Autodesk Fusion 360 part; units mm, degrees
(part 4 of 13)
sketch "Sketch30" plane through (0, 0, 9) normal (0, 0, 1) x (-1, 0, 0)
  line L0 (-20, -24.98) -> (-20, -25.98)
  line L1 (-20, -25.98) -> (-21, -25.98)
  line L2 (-21, -25.98) -> (-21, -24.98)
  line L3 (-21, -24.98) -> (-20, -24.98)
  line L4 (-23, -24.98) -> (-23, -25.98)
  line L5 (-23, -25.98) -> (-24, -25.98)
  line L6 (-24, -25.98) -> (-24, -24.98)
  line L7 (-24, -24.98) -> (-23, -24.98)
  line L8 (-20, -27.61) -> (-20, -28.61)
  line L9 (-20, -28.61) -> (-21, -28.61)
  line L10 (-21, -28.61) -> (-21, -27.61)
  line L11 (-21, -27.61) -> (-20, -27.61)
  line L12 (-23, -27.61) -> (-23, -28.61)
  line L13 (-23, -28.61) -> (-24, -28.61)
  line L14 (-24, -28.61) -> (-24, -27.61)
  line L15 (-24, -27.61) -> (-23, -27.61)
  line L16 (-20, -30.24) -> (-20, -31.24)
  line L17 (-20, -31.24) -> (-21, -31.24)
  line L18 (-21, -31.24) -> (-21, -30.24)
  line L19 (-21, -30.24) -> (-20, -30.24)
  line L20 (-23, -30.24) -> (-23, -31.24)
  line L21 (-23, -31.24) -> (-24, -31.24)
  line L22 (-24, -31.24) -> (-24, -30.24)
  line L23 (-24, -30.24) -> (-23, -30.24)
  line L24 (-20, -32.87) -> (-20, -33.87)
  line L25 (-20, -33.87) -> (-21, -33.87)
  line L26 (-21, -33.87) -> (-21, -32.87)
  line L27 (-21, -32.87) -> (-20, -32.87)
  line L28 (-23, -32.87) -> (-23, -33.87)
  line L29 (-23, -33.87) -> (-24, -33.87)
  line L30 (-24, -33.87) -> (-24, -32.87)
  line L31 (-24, -32.87) -> (-23, -32.87)
  line L32 (-20, -35.5) -> (-20, -36.5)
  line L33 (-20, -36.5) -> (-21, -36.5)
  line L34 (-21, -36.5) -> (-21, -35.5)
  line L35 (-21, -35.5) -> (-20, -35.5)
  line L36 (-23, -35.5) -> (-23, -36.5)
  line L37 (-23, -36.5) -> (-24, -36.5)
  line L38 (-24, -36.5) -> (-24, -35.5)
  line L39 (-24, -35.5) -> (-23, -35.5)
  line L40 (-13.7, 38.77) -> (-13.7, 37.77)
  line L41 (-13.7, 37.77) -> (-14.7, 37.77)
  line L42 (-14.7, 37.77) -> (-14.7, 38.77)
  line L43 (-14.7, 38.77) -> (-13.7, 38.77)
  line L44 (-13.7, 36.14) -> (-13.7, 35.14)
  line L45 (-13.7, 35.14) -> (-14.7, 35.14)
  line L46 (-14.7, 35.14) -> (-14.7, 36.14)
  line L47 (-14.7, 36.14) -> (-13.7, 36.14)
  line L48 (-13.7, 33.51) -> (-13.7, 32.51)
  line L49 (-13.7, 32.51) -> (-14.7, 32.51)
  line L50 (-14.7, 32.51) -> (-14.7, 33.51)
  line L51 (-14.7, 33.51) -> (-13.7, 33.51)
  line L52 (-13.7, 30.88) -> (-13.7, 29.88)
  line L53 (-13.7, 29.88) -> (-14.7, 29.88)
  line L54 (-14.7, 29.88) -> (-14.7, 30.88)
  line L55 (-14.7, 30.88) -> (-13.7, 30.88)
  line L56 (-13.7, 28.25) -> (-13.7, 27.25)
  line L57 (-13.7, 27.25) -> (-14.7, 27.25)
  line L58 (-14.7, 27.25) -> (-14.7, 28.25)
  line L59 (-14.7, 28.25) -> (-13.7, 28.25)
  line L60 (-13.7, 25.62) -> (-13.7, 24.62)
  line L61 (-13.7, 24.62) -> (-14.7, 24.62)
  line L62 (-14.7, 24.62) -> (-14.7, 25.62)
  line L63 (-14.7, 25.62) -> (-13.7, 25.62)
  line L64 (-13.7, 22.99) -> (-13.7, 21.99)
  line L65 (-13.7, 21.99) -> (-14.7, 21.99)
  line L66 (-14.7, 21.99) -> (-14.7, 22.99)
  line L67 (-14.7, 22.99) -> (-13.7, 22.99)
  line L68 (-13.7, 20.36) -> (-13.7, 19.36)
  line L69 (-13.7, 19.36) -> (-14.7, 19.36)
  line L70 (-14.7, 19.36) -> (-14.7, 20.36)
  line L71 (-14.7, 20.36) -> (-13.7, 20.36)
  line L72 (-13.7, 17.73) -> (-13.7, 16.73)
  line L73 (-13.7, 16.73) -> (-14.7, 16.73)
  line L74 (-14.7, 16.73) -> (-14.7, 17.73)
  line L75 (-14.7, 17.73) -> (-13.7, 17.73)
  line L76 (-13.7, 15.1) -> (-13.7, 14.1)
  line L77 (-13.7, 14.1) -> (-14.7, 14.1)
  line L78 (-14.7, 14.1) -> (-14.7, 15.1)
  line L79 (-14.7, 15.1) -> (-13.7, 15.1)
  line L80 (-13.7, 12.47) -> (-13.7, 11.47)
  line L81 (-13.7, 11.47) -> (-14.7, 11.47)
  line L82 (-14.7, 11.47) -> (-14.7, 12.47)
  line L83 (-14.7, 12.47) -> (-13.7, 12.47)
  line L84 (-13.7, 9.84) -> (-13.7, 8.84)
  line L85 (-13.7, 8.84) -> (-14.7, 8.84)
  line L86 (-14.7, 8.84) -> (-14.7, 9.84)
  line L87 (-14.7, 9.84) -> (-13.7, 9.84)
  line L88 (-13.7, 7.21) -> (-13.7, 6.21)
  line L89 (-13.7, 6.21) -> (-14.7, 6.21)
  line L90 (-14.7, 6.21) -> (-14.7, 7.21)
  line L91 (-14.7, 7.21) -> (-13.7, 7.21)
  line L92 (-13.7, 4.58) -> (-13.7, 3.58)
  line L93 (-13.7, 3.58) -> (-14.7, 3.58)
  line L94 (-14.7, 3.58) -> (-14.7, 4.58)
  line L95 (-14.7, 4.58) -> (-13.7, 4.58)
  line L96 (-13.7, 1.95) -> (-13.7, 0.95)
  line L97 (-13.7, 0.95) -> (-14.7, 0.95)
  line L98 (-14.7, 0.95) -> (-14.7, 1.95)
  line L99 (-14.7, 1.95) -> (-13.7, 1.95)
  line L100 (-13.7, -0.68) -> (-13.7, -1.68)
  line L101 (-13.7, -1.68) -> (-14.7, -1.68)
  line L102 (-14.7, -1.68) -> (-14.7, -0.68)
  line L103 (-14.7, -0.68) -> (-13.7, -0.68)
  line L104 (-13.7, -3.31) -> (-13.7, -4.31)
  line L105 (-13.7, -4.31) -> (-14.7, -4.31)
  line L106 (-14.7, -4.31) -> (-14.7, -3.31)
  line L107 (-14.7, -3.31) -> (-13.7, -3.31)
  line L108 (-13.7, -5.94) -> (-13.7, -6.94)
  line L109 (-13.7, -6.94) -> (-14.7, -6.94)
  line L110 (-14.7, -6.94) -> (-14.7, -5.94)
  line L111 (-14.7, -5.94) -> (-13.7, -5.94)
  line L112 (-13.7, -8.57) -> (-13.7, -9.57)
  line L113 (-13.7, -9.57) -> (-14.7, -9.57)
  line L114 (-14.7, -9.57) -> (-14.7, -8.57)
  line L115 (-14.7, -8.57) -> (-13.7, -8.57)
  line L116 (-13.7, -11.2) -> (-13.7, -12.2)
  line L117 (-13.7, -12.2) -> (-14.7, -12.2)
  line L118 (-14.7, -12.2) -> (-14.7, -11.2)
  line L119 (-14.7, -11.2) -> (-13.7, -11.2)
  line L120 (-13.7, -13.83) -> (-13.7, -14.83)
  line L121 (-13.7, -14.83) -> (-14.7, -14.83)
  line L122 (-14.7, -14.83) -> (-14.7, -13.83)
  line L123 (-14.7, -13.83) -> (-13.7, -13.83)
  line L124 (-13.7, -16.46) -> (-13.7, -17.46)
  line L125 (-13.7, -17.46) -> (-14.7, -17.46)
  line L126 (-14.7, -17.46) -> (-14.7, -16.46)
  line L127 (-14.7, -16.46) -> (-13.7, -16.46)
  line L128 (-13.7, -19.09) -> (-13.7, -20.09)
  line L129 (-13.7, -20.09) -> (-14.7, -20.09)
  line L130 (-14.7, -20.09) -> (-14.7, -19.09)
  line L131 (-14.7, -19.09) -> (-13.7, -19.09)
  line L132 (-13.7, -21.72) -> (-13.7, -22.72)
  line L133 (-13.7, -22.72) -> (-14.7, -22.72)
  line L134 (-14.7, -22.72) -> (-14.7, -21.72)
  line L135 (-14.7, -21.72) -> (-13.7, -21.72)
  line L136 (-13.7, -24.35) -> (-13.7, -25.35)
  line L137 (-13.7, -25.35) -> (-14.7, -25.35)
  line L138 (-14.7, -25.35) -> (-14.7, -24.35)
  line L139 (-14.7, -24.35) -> (-13.7, -24.35)
  line L140 (-13.7, -26.98) -> (-13.7, -27.98)
  line L141 (-13.7, -27.98) -> (-14.7, -27.98)
  line L142 (-14.7, -27.98) -> (-14.7, -26.98)
  line L143 (-14.7, -26.98) -> (-13.7, -26.98)
  line L144 (-13.7, -29.61) -> (-13.7, -30.61)
  line L145 (-13.7, -30.61) -> (-14.7, -30.61)
  line L146 (-14.7, -30.61) -> (-14.7, -29.61)
  line L147 (-14.7, -29.61) -> (-13.7, -29.61)
  line L148 (-13.7, -32.24) -> (-13.7, -33.24)
  line L149 (-13.7, -33.24) -> (-14.7, -33.24)
  line L150 (-14.7, -33.24) -> (-14.7, -32.24)
  line L151 (-14.7, -32.24) -> (-13.7, -32.24)
  line L152 (-13.7, -34.87) -> (-13.7, -35.87)
  line L153 (-13.7, -35.87) -> (-14.7, -35.87)
  line L154 (-14.7, -35.87) -> (-14.7, -34.87)
  line L155 (-14.7, -34.87) -> (-13.7, -34.87)
  line L156 (-13.7, -37.5) -> (-13.7, -38.5)
  line L157 (-13.7, -38.5) -> (-14.7, -38.5)
  line L158 (-14.7, -38.5) -> (-14.7, -37.5)
  line L159 (-14.7, -37.5) -> (-13.7, -37.5)
  line L160 (-10.9, 38.77) -> (-10.9, 37.77)
  line L161 (-10.9, 37.77) -> (-11.9, 37.77)
  line L162 (-11.9, 37.77) -> (-11.9, 38.77)
  line L163 (-11.9, 38.77) -> (-10.9, 38.77)
  line L164 (-10.9, 36.14) -> (-10.9, 35.14)
  line L165 (-10.9, 35.14) -> (-11.9, 35.14)
  line L166 (-11.9, 35.14) -> (-11.9, 36.14)
  line L167 (-11.9, 36.14) -> (-10.9, 36.14)
  line L168 (-10.9, 33.51) -> (-10.9, 32.51)
  line L169 (-10.9, 32.51) -> (-11.9, 32.51)
  line L170 (-11.9, 32.51) -> (-11.9, 33.51)
  line L171 (-11.9, 33.51) -> (-10.9, 33.51)
  line L172 (-10.9, 30.88) -> (-10.9, 29.88)
  line L173 (-10.9, 29.88) -> (-11.9, 29.88)
  line L174 (-11.9, 29.88) -> (-11.9, 30.88)
  line L175 (-11.9, 30.88) -> (-10.9, 30.88)
  line L176 (-10.9, 28.25) -> (-10.9, 27.25)
  line L177 (-10.9, 27.25) -> (-11.9, 27.25)
  line L178 (-11.9, 27.25) -> (-11.9, 28.25)
  line L179 (-11.9, 28.25) -> (-10.9, 28.25)
  line L180 (-10.9, 25.62) -> (-10.9, 24.62)
  line L181 (-10.9, 24.62) -> (-11.9, 24.62)
  line L182 (-11.9, 24.62) -> (-11.9, 25.62)
  line L183 (-11.9, 25.62) -> (-10.9, 25.62)
  line L184 (-10.9, 22.99) -> (-10.9, 21.99)
  line L185 (-10.9, 21.99) -> (-11.9, 21.99)
  line L186 (-11.9, 21.99) -> (-11.9, 22.99)
  line L187 (-11.9, 22.99) -> (-10.9, 22.99)
  line L188 (-10.9, 20.36) -> (-10.9, 19.36)
  line L189 (-10.9, 19.36) -> (-11.9, 19.36)
  line L190 (-11.9, 19.36) -> (-11.9, 20.36)
  line L191 (-11.9, 20.36) -> (-10.9, 20.36)
  line L192 (-10.9, 17.73) -> (-10.9, 16.73)
  line L193 (-10.9, 16.73) -> (-11.9, 16.73)
  line L194 (-11.9, 16.73) -> (-11.9, 17.73)
  line L195 (-11.9, 17.73) -> (-10.9, 17.73)
  line L196 (-10.9, 15.1) -> (-10.9, 14.1)
  line L197 (-10.9, 14.1) -> (-11.9, 14.1)
  line L198 (-11.9, 14.1) -> (-11.9, 15.1)
  line L199 (-11.9, 15.1) -> (-10.9, 15.1)
  line L200 (-10.9, 12.47) -> (-10.9, 11.47)
  line L201 (-10.9, 11.47) -> (-11.9, 11.47)
  line L202 (-11.9, 11.47) -> (-11.9, 12.47)
  line L203 (-11.9, 12.47) -> (-10.9, 12.47)
  line L204 (-10.9, 9.84) -> (-10.9, 8.84)
  line L205 (-10.9, 8.84) -> (-11.9, 8.84)
  line L206 (-11.9, 8.84) -> (-11.9, 9.84)
  line L207 (-11.9, 9.84) -> (-10.9, 9.84)
  line L208 (-10.9, 7.21) -> (-10.9, 6.21)
  line L209 (-10.9, 6.21) -> (-11.9, 6.21)
  line L210 (-11.9, 6.21) -> (-11.9, 7.21)
  line L211 (-11.9, 7.21) -> (-10.9, 7.21)
  line L212 (-10.9, 4.58) -> (-10.9, 3.58)
  line L213 (-10.9, 3.58) -> (-11.9, 3.58)
  line L214 (-11.9, 3.58) -> (-11.9, 4.58)
  line L215 (-11.9, 4.58) -> (-10.9, 4.58)
  line L216 (-10.9, 1.95) -> (-10.9, 0.95)
  line L217 (-10.9, 0.95) -> (-11.9, 0.95)
  line L218 (-11.9, 0.95) -> (-11.9, 1.95)
  line L219 (-11.9, 1.95) -> (-10.9, 1.95)
  line L220 (-10.9, -0.68) -> (-10.9, -1.68)
  line L221 (-10.9, -1.68) -> (-11.9, -1.68)
  line L222 (-11.9, -1.68) -> (-11.9, -0.68)
  line L223 (-11.9, -0.68) -> (-10.9, -0.68)
  line L224 (-10.9, -3.31) -> (-10.9, -4.31)
  line L225 (-10.9, -4.31) -> (-11.9, -4.31)
  line L226 (-11.9, -4.31) -> (-11.9, -3.31)
  line L227 (-11.9, -3.31) -> (-10.9, -3.31)
  line L228 (-10.9, -5.94) -> (-10.9, -6.94)
  line L229 (-10.9, -6.94) -> (-11.9, -6.94)
  line L230 (-11.9, -6.94) -> (-11.9, -5.94)
  line L231 (-11.9, -5.94) -> (-10.9, -5.94)
  line L232 (-10.9, -8.57) -> (-10.9, -9.57)
  line L233 (-10.9, -9.57) -> (-11.9, -9.57)
  line L234 (-11.9, -9.57) -> (-11.9, -8.57)
  line L235 (-11.9, -8.57) -> (-10.9, -8.57)
  line L236 (-10.9, -11.2) -> (-10.9, -12.2)
  line L237 (-10.9, -12.2) -> (-11.9, -12.2)
  line L238 (-11.9, -12.2) -> (-11.9, -11.2)
  line L239 (-11.9, -11.2) -> (-10.9, -11.2)
  line L240 (-10.9, -13.83) -> (-10.9, -14.83)
  line L241 (-10.9, -14.83) -> (-11.9, -14.83)
  line L242 (-11.9, -14.83) -> (-11.9, -13.83)
  line L243 (-11.9, -13.83) -> (-10.9, -13.83)
  line L244 (-10.9, -16.46) -> (-10.9, -17.46)
  line L245 (-10.9, -17.46) -> (-11.9, -17.46)
  line L246 (-11.9, -17.46) -> (-11.9, -16.46)
  line L247 (-11.9, -16.46) -> (-10.9, -16.46)
  line L248 (-10.9, -19.09) -> (-10.9, -20.09)
  line L249 (-10.9, -20.09) -> (-11.9, -20.09)
  line L250 (-11.9, -20.09) -> (-11.9, -19.09)
  line L251 (-11.9, -19.09) -> (-10.9, -19.09)
  line L252 (-10.9, -21.72) -> (-10.9, -22.72)
  line L253 (-10.9, -22.72) -> (-11.9, -22.72)
  line L254 (-11.9, -22.72) -> (-11.9, -21.72)
  line L255 (-11.9, -21.72) -> (-10.9, -21.72)
  line L256 (-10.9, -24.35) -> (-10.9, -25.35)
  line L257 (-10.9, -25.35) -> (-11.9, -25.35)
  line L258 (-11.9, -25.35) -> (-11.9, -24.35)
  line L259 (-11.9, -24.35) -> (-10.9, -24.35)
  line L260 (-10.9, -26.98) -> (-10.9, -27.98)
  line L261 (-10.9, -27.98) -> (-11.9, -27.98)
  line L262 (-11.9, -27.98) -> (-11.9, -26.98)
  line L263 (-11.9, -26.98) -> (-10.9, -26.98)
  line L264 (-10.9, -29.61) -> (-10.9, -30.61)
  line L265 (-10.9, -30.61) -> (-11.9, -30.61)
  line L266 (-11.9, -30.61) -> (-11.9, -29.61)
  line L267 (-11.9, -29.61) -> (-10.9, -29.61)
  line L268 (-10.9, -32.24) -> (-10.9, -33.24)
  line L269 (-10.9, -33.24) -> (-11.9, -33.24)
  line L270 (-11.9, -33.24) -> (-11.9, -32.24)
  line L271 (-11.9, -32.24) -> (-10.9, -32.24)
  line L272 (-10.9, -34.87) -> (-10.9, -35.87)
  line L273 (-10.9, -35.87) -> (-11.9, -35.87)
  line L274 (-11.9, -35.87) -> (-11.9, -34.87)
  line L275 (-11.9, -34.87) -> (-10.9, -34.87)
  line L276 (-10.9, -37.5) -> (-10.9, -38.5)
  line L277 (-10.9, -38.5) -> (-11.9, -38.5)
  line L278 (-11.9, -38.5) -> (-11.9, -37.5)
  line L279 (-11.9, -37.5) -> (-10.9, -37.5)
  line L280 (-8.1, 38.77) -> (-8.1, 37.77)
  line L281 (-8.1, 37.77) -> (-9.1, 37.77)
  line L282 (-9.1, 37.77) -> (-9.1, 38.77)
  line L283 (-9.1, 38.77) -> (-8.1, 38.77)
  line L284 (-8.1, 36.14) -> (-8.1, 35.14)
  line L285 (-8.1, 35.14) -> (-9.1, 35.14)
  line L286 (-9.1, 35.14) -> (-9.1, 36.14)
  line L287 (-9.1, 36.14) -> (-8.1, 36.14)
  line L288 (-8.1, 33.51) -> (-8.1, 32.51)
  line L289 (-8.1, 32.51) -> (-9.1, 32.51)
  line L290 (-9.1, 32.51) -> (-9.1, 33.51)
  line L291 (-9.1, 33.51) -> (-8.1, 33.51)
  line L292 (-8.1, 30.88) -> (-8.1, 29.88)
  line L293 (-8.1, 29.88) -> (-9.1, 29.88)
  line L294 (-9.1, 29.88) -> (-9.1, 30.88)
  line L295 (-9.1, 30.88) -> (-8.1, 30.88)
  line L296 (-8.1, 28.25) -> (-8.1, 27.25)
  line L297 (-8.1, 27.25) -> (-9.1, 27.25)
  line L298 (-9.1, 27.25) -> (-9.1, 28.25)
  line L299 (-9.1, 28.25) -> (-8.1, 28.25)
  line L300 (-8.1, 25.62) -> (-8.1, 24.62)
  line L301 (-8.1, 24.62) -> (-9.1, 24.62)
  line L302 (-9.1, 24.62) -> (-9.1, 25.62)
  line L303 (-9.1, 25.62) -> (-8.1, 25.62)
  line L304 (-8.1, 22.99) -> (-8.1, 21.99)
  line L305 (-8.1, 21.99) -> (-9.1, 21.99)
  line L306 (-9.1, 21.99) -> (-9.1, 22.99)
  line L307 (-9.1, 22.99) -> (-8.1, 22.99)
  line L308 (-8.1, 20.36) -> (-8.1, 19.36)
  line L309 (-8.1, 19.36) -> (-9.1, 19.36)
  line L310 (-9.1, 19.36) -> (-9.1, 20.36)
  line L311 (-9.1, 20.36) -> (-8.1, 20.36)
  line L312 (-8.1, 17.73) -> (-8.1, 16.73)
  line L313 (-8.1, 16.73) -> (-9.1, 16.73)
  line L314 (-9.1, 16.73) -> (-9.1, 17.73)
  line L315 (-9.1, 17.73) -> (-8.1, 17.73)
  line L316 (-8.1, 15.1) -> (-8.1, 14.1)
  line L317 (-8.1, 14.1) -> (-9.1, 14.1)
  line L318 (-9.1, 14.1) -> (-9.1, 15.1)
  line L319 (-9.1, 15.1) -> (-8.1, 15.1)
  line L320 (-8.1, 12.47) -> (-8.1, 11.47)
  line L321 (-8.1, 11.47) -> (-9.1, 11.47)
  line L322 (-9.1, 11.47) -> (-9.1, 12.47)
  line L323 (-9.1, 12.47) -> (-8.1, 12.47)
  line L324 (-8.1, 9.84) -> (-8.1, 8.84)
  line L325 (-8.1, 8.84) -> (-9.1, 8.84)
  line L326 (-9.1, 8.84) -> (-9.1, 9.84)
  line L327 (-9.1, 9.84) -> (-8.1, 9.84)
  line L328 (-8.1, 7.21) -> (-8.1, 6.21)
  line L329 (-8.1, 6.21) -> (-9.1, 6.21)
  line L330 (-9.1, 6.21) -> (-9.1, 7.21)
  line L331 (-9.1, 7.21) -> (-8.1, 7.21)
  line L332 (-8.1, 4.58) -> (-8.1, 3.58)
  line L333 (-8.1, 3.58) -> (-9.1, 3.58)
  line L334 (-9.1, 3.58) -> (-9.1, 4.58)
  line L335 (-9.1, 4.58) -> (-8.1, 4.58)
  line L336 (-8.1, 1.95) -> (-8.1, 0.95)
  line L337 (-8.1, 0.95) -> (-9.1, 0.95)
  line L338 (-9.1, 0.95) -> (-9.1, 1.95)
  line L339 (-9.1, 1.95) -> (-8.1, 1.95)
  line L340 (-8.1, -0.68) -> (-8.1, -1.68)
  line L341 (-8.1, -1.68) -> (-9.1, -1.68)
  line L342 (-9.1, -1.68) -> (-9.1, -0.68)
  line L343 (-9.1, -0.68) -> (-8.1, -0.68)
  line L344 (-8.1, -3.31) -> (-8.1, -4.31)
  line L345 (-8.1, -4.31) -> (-9.1, -4.31)
  line L346 (-9.1, -4.31) -> (-9.1, -3.31)
  line L347 (-9.1, -3.31) -> (-8.1, -3.31)
  line L348 (-8.1, -5.94) -> (-8.1, -6.94)
  line L349 (-8.1, -6.94) -> (-9.1, -6.94)
  line L350 (-9.1, -6.94) -> (-9.1, -5.94)
  line L351 (-9.1, -5.94) -> (-8.1, -5.94)
  line L352 (-8.1, -8.57) -> (-8.1, -9.57)
  line L353 (-8.1, -9.57) -> (-9.1, -9.57)
  line L354 (-9.1, -9.57) -> (-9.1, -8.57)
  line L355 (-9.1, -8.57) -> (-8.1, -8.57)
  line L356 (-8.1, -11.2) -> (-8.1, -12.2)
  line L357 (-8.1, -12.2) -> (-9.1, -12.2)
  line L358 (-9.1, -12.2) -> (-9.1, -11.2)
  line L359 (-9.1, -11.2) -> (-8.1, -11.2)
  line L360 (-8.1, -13.83) -> (-8.1, -14.83)
  line L361 (-8.1, -14.83) -> (-9.1, -14.83)
  line L362 (-9.1, -14.83) -> (-9.1, -13.83)
  line L363 (-9.1, -13.83) -> (-8.1, -13.83)
  line L364 (-8.1, -16.46) -> (-8.1, -17.46)
  line L365 (-8.1, -17.46) -> (-9.1, -17.46)
  line L366 (-9.1, -17.46) -> (-9.1, -16.46)
  line L367 (-9.1, -16.46) -> (-8.1, -16.46)
  line L368 (-8.1, -19.09) -> (-8.1, -20.09)
  line L369 (-8.1, -20.09) -> (-9.1, -20.09)
  line L370 (-9.1, -20.09) -> (-9.1, -19.09)
  line L371 (-9.1, -19.09) -> (-8.1, -19.09)
  line L372 (-8.1, -21.72) -> (-8.1, -22.72)
  line L373 (-8.1, -22.72) -> (-9.1, -22.72)
  line L374 (-9.1, -22.72) -> (-9.1, -21.72)
  line L375 (-9.1, -21.72) -> (-8.1, -21.72)
  line L376 (-8.1, -24.35) -> (-8.1, -25.35)
  line L377 (-8.1, -25.35) -> (-9.1, -25.35)
  line L378 (-9.1, -25.35) -> (-9.1, -24.35)
  line L379 (-9.1, -24.35) -> (-8.1, -24.35)
  line L380 (-8.1, -26.98) -> (-8.1, -27.98)
  line L381 (-8.1, -27.98) -> (-9.1, -27.98)
  line L382 (-9.1, -27.98) -> (-9.1, -26.98)
  line L383 (-9.1, -26.98) -> (-8.1, -26.98)
  line L384 (-8.1, -29.61) -> (-8.1, -30.61)
  line L385 (-8.1, -30.61) -> (-9.1, -30.61)
  line L386 (-9.1, -30.61) -> (-9.1, -29.61)
  line L387 (-9.1, -29.61) -> (-8.1, -29.61)
  line L388 (-8.1, -32.24) -> (-8.1, -33.24)
  line L389 (-8.1, -33.24) -> (-9.1, -33.24)
  line L390 (-9.1, -33.24) -> (-9.1, -32.24)
  line L391 (-9.1, -32.24) -> (-8.1, -32.24)
  line L392 (-8.1, -34.87) -> (-8.1, -35.87)
  line L393 (-8.1, -35.87) -> (-9.1, -35.87)
  line L394 (-9.1, -35.87) -> (-9.1, -34.87)
  line L395 (-9.1, -34.87) -> (-8.1, -34.87)
  line L396 (-8.1, -37.5) -> (-8.1, -38.5)
  line L397 (-8.1, -38.5) -> (-9.1, -38.5)
  line L398 (-9.1, -38.5) -> (-9.1, -37.5)
  line L399 (-9.1, -37.5) -> (-8.1, -37.5)
  line L400 (-5.3, 38.77) -> (-5.3, 37.77)
  line L401 (-5.3, 37.77) -> (-6.3, 37.77)
  line L402 (-6.3, 37.77) -> (-6.3, 38.77)
  line L403 (-6.3, 38.77) -> (-5.3, 38.77)
  line L404 (-5.3, 36.14) -> (-5.3, 35.14)
  line L405 (-5.3, 35.14) -> (-6.3, 35.14)
  line L406 (-6.3, 35.14) -> (-6.3, 36.14)
  line L407 (-6.3, 36.14) -> (-5.3, 36.14)
  line L408 (-5.3, 33.51) -> (-5.3, 32.51)
  line L409 (-5.3, 32.51) -> (-6.3, 32.51)
  line L410 (-6.3, 32.51) -> (-6.3, 33.51)
  line L411 (-6.3, 33.51) -> (-5.3, 33.51)
  line L412 (-5.3, 30.88) -> (-5.3, 29.88)
  line L413 (-5.3, 29.88) -> (-6.3, 29.88)
  line L414 (-6.3, 29.88) -> (-6.3, 30.88)
  line L415 (-6.3, 30.88) -> (-5.3, 30.88)
  line L416 (-5.3, 28.25) -> (-5.3, 27.25)
  line L417 (-5.3, 27.25) -> (-6.3, 27.25)
  line L418 (-6.3, 27.25) -> (-6.3, 28.25)
  line L419 (-6.3, 28.25) -> (-5.3, 28.25)
  line L420 (-5.3, 25.62) -> (-5.3, 24.62)
  line L421 (-5.3, 24.62) -> (-6.3, 24.62)
  line L422 (-6.3, 24.62) -> (-6.3, 25.62)
  line L423 (-6.3, 25.62) -> (-5.3, 25.62)
  line L424 (-5.3, 22.99) -> (-5.3, 21.99)
  line L425 (-5.3, 21.99) -> (-6.3, 21.99)
  line L426 (-6.3, 21.99) -> (-6.3, 22.99)
  line L427 (-6.3, 22.99) -> (-5.3, 22.99)
  line L428 (-5.3, 20.36) -> (-5.3, 19.36)
  line L429 (-5.3, 19.36) -> (-6.3, 19.36)
  line L430 (-6.3, 19.36) -> (-6.3, 20.36)
  line L431 (-6.3, 20.36) -> (-5.3, 20.36)
  line L432 (-5.3, 17.73) -> (-5.3, 16.73)
  line L433 (-5.3, 16.73) -> (-6.3, 16.73)
  line L434 (-6.3, 16.73) -> (-6.3, 17.73)
  line L435 (-6.3, 17.73) -> (-5.3, 17.73)
  line L436 (-5.3, 15.1) -> (-5.3, 14.1)
  line L437 (-5.3, 14.1) -> (-6.3, 14.1)
  line L438 (-6.3, 14.1) -> (-6.3, 15.1)
  line L439 (-6.3, 15.1) -> (-5.3, 15.1)
  line L440 (-5.3, 12.47) -> (-5.3, 11.47)
  line L441 (-5.3, 11.47) -> (-6.3, 11.47)
  line L442 (-6.3, 11.47) -> (-6.3, 12.47)
  line L443 (-6.3, 12.47) -> (-5.3, 12.47)
  line L444 (-5.3, 9.84) -> (-5.3, 8.84)
  line L445 (-5.3, 8.84) -> (-6.3, 8.84)
  line L446 (-6.3, 8.84) -> (-6.3, 9.84)
  line L447 (-6.3, 9.84) -> (-5.3, 9.84)
  line L448 (-5.3, 7.21) -> (-5.3, 6.21)
  line L449 (-5.3, 6.21) -> (-6.3, 6.21)
  line L450 (-6.3, 6.21) -> (-6.3, 7.21)
  line L451 (-6.3, 7.21) -> (-5.3, 7.21)
  line L452 (-5.3, 4.58) -> (-5.3, 3.58)
  line L453 (-5.3, 3.58) -> (-6.3, 3.58)
  line L454 (-6.3, 3.58) -> (-6.3, 4.58)
  line L455 (-6.3, 4.58) -> (-5.3, 4.58)
  line L456 (-5.3, 1.95) -> (-5.3, 0.95)
  line L457 (-5.3, 0.95) -> (-6.3, 0.95)
  line L458 (-6.3, 0.95) -> (-6.3, 1.95)
  line L459 (-6.3, 1.95) -> (-5.3, 1.95)
  line L460 (-5.3, -0.68) -> (-5.3, -1.68)
  line L461 (-5.3, -1.68) -> (-6.3, -1.68)
  line L462 (-6.3, -1.68) -> (-6.3, -0.68)
  line L463 (-6.3, -0.68) -> (-5.3, -0.68)
  line L464 (-5.3, -3.31) -> (-5.3, -4.31)
  line L465 (-5.3, -4.31) -> (-6.3, -4.31)
  line L466 (-6.3, -4.31) -> (-6.3, -3.31)
  line L467 (-6.3, -3.31) -> (-5.3, -3.31)
  line L468 (-5.3, -5.94) -> (-5.3, -6.94)
  line L469 (-5.3, -6.94) -> (-6.3, -6.94)
  line L470 (-6.3, -6.94) -> (-6.3, -5.94)
  line L471 (-6.3, -5.94) -> (-5.3, -5.94)
  line L472 (-5.3, -8.57) -> (-5.3, -9.57)
  line L473 (-5.3, -9.57) -> (-6.3, -9.57)
  line L474 (-6.3, -9.57) -> (-6.3, -8.57)
  line L475 (-6.3, -8.57) -> (-5.3, -8.57)
  line L476 (-5.3, -11.2) -> (-5.3, -12.2)
  line L477 (-5.3, -12.2) -> (-6.3, -12.2)
  line L478 (-6.3, -12.2) -> (-6.3, -11.2)
  line L479 (-6.3, -11.2) -> (-5.3, -11.2)
  line L480 (-5.3, -13.83) -> (-5.3, -14.83)
  line L481 (-5.3, -14.83) -> (-6.3, -14.83)
  line L482 (-6.3, -14.83) -> (-6.3, -13.83)
  line L483 (-6.3, -13.83) -> (-5.3, -13.83)
  line L484 (-5.3, -16.46) -> (-5.3, -17.46)
  line L485 (-5.3, -17.46) -> (-6.3, -17.46)
  line L486 (-6.3, -17.46) -> (-6.3, -16.46)
  line L487 (-6.3, -16.46) -> (-5.3, -16.46)
  line L488 (-5.3, -19.09) -> (-5.3, -20.09)
  line L489 (-5.3, -20.09) -> (-6.3, -20.09)
  line L490 (-6.3, -20.09) -> (-6.3, -19.09)
  line L491 (-6.3, -19.09) -> (-5.3, -19.09)
  line L492 (-5.3, -21.72) -> (-5.3, -22.72)
  line L493 (-5.3, -22.72) -> (-6.3, -22.72)
  line L494 (-6.3, -22.72) -> (-6.3, -21.72)
  line L495 (-6.3, -21.72) -> (-5.3, -21.72)
  line L496 (-5.3, -24.35) -> (-5.3, -25.35)
  line L497 (-5.3, -25.35) -> (-6.3, -25.35)
  line L498 (-6.3, -25.35) -> (-6.3, -24.35)
  line L499 (-6.3, -24.35) -> (-5.3, -24.35)
  line L500 (-5.3, -26.98) -> (-5.3, -27.98)
  line L501 (-5.3, -27.98) -> (-6.3, -27.98)
  line L502 (-6.3, -27.98) -> (-6.3, -26.98)
  line L503 (-6.3, -26.98) -> (-5.3, -26.98)
  line L504 (-5.3, -29.61) -> (-5.3, -30.61)
  line L505 (-5.3, -30.61) -> (-6.3, -30.61)
  line L506 (-6.3, -30.61) -> (-6.3, -29.61)
  line L507 (-6.3, -29.61) -> (-5.3, -29.61)
  line L508 (-5.3, -32.24) -> (-5.3, -33.24)
  line L509 (-5.3, -33.24) -> (-6.3, -33.24)
  line L510 (-6.3, -33.24) -> (-6.3, -32.24)
  line L511 (-6.3, -32.24) -> (-5.3, -32.24)
  line L512 (-5.3, -34.87) -> (-5.3, -35.87)
  line L513 (-5.3, -35.87) -> (-6.3, -35.87)
  line L514 (-6.3, -35.87) -> (-6.3, -34.87)
  line L515 (-6.3, -34.87) -> (-5.3, -34.87)
  line L516 (-5.3, -37.5) -> (-5.3, -38.5)
  line L517 (-5.3, -38.5) -> (-6.3, -38.5)
  line L518 (-6.3, -38.5) -> (-6.3, -37.5)
  line L519 (-6.3, -37.5) -> (-5.3, -37.5)
  line L520 (-2.5, 38.77) -> (-2.5, 37.77)
  line L521 (-2.5, 37.77) -> (-3.5, 37.77)
  line L522 (-3.5, 37.77) -> (-3.5, 38.77)
  line L523 (-3.5, 38.77) -> (-2.5, 38.77)
  line L524 (-2.5, 36.14) -> (-2.5, 35.14)
  line L525 (-2.5, 35.14) -> (-3.5, 35.14)
  line L526 (-3.5, 35.14) -> (-3.5, 36.14)
  line L527 (-3.5, 36.14) -> (-2.5, 36.14)
  line L528 (-2.5, 33.51) -> (-2.5, 32.51)
  line L529 (-2.5, 32.51) -> (-3.5, 32.51)
  line L530 (-3.5, 32.51) -> (-3.5, 33.51)
  line L531 (-3.5, 33.51) -> (-2.5, 33.51)
  line L532 (-2.5, 30.88) -> (-2.5, 29.88)
  line L533 (-2.5, 29.88) -> (-3.5, 29.88)
  line L534 (-3.5, 29.88) -> (-3.5, 30.88)
  line L535 (-3.5, 30.88) -> (-2.5, 30.88)
  line L536 (-2.5, 28.25) -> (-2.5, 27.25)
  line L537 (-2.5, 27.25) -> (-3.5, 27.25)
  line L538 (-3.5, 27.25) -> (-3.5, 28.25)
  line L539 (-3.5, 28.25) -> (-2.5, 28.25)
  line L540 (-2.5, 25.62) -> (-2.5, 24.62)
  line L541 (-2.5, 24.62) -> (-3.5, 24.62)
  line L542 (-3.5, 24.62) -> (-3.5, 25.62)
  line L543 (-3.5, 25.62) -> (-2.5, 25.62)
  line L544 (-2.5, 22.99) -> (-2.5, 21.99)
  line L545 (-2.5, 21.99) -> (-3.5, 21.99)
  line L546 (-3.5, 21.99) -> (-3.5, 22.99)
  line L547 (-3.5, 22.99) -> (-2.5, 22.99)
  line L548 (-2.5, 20.36) -> (-2.5, 19.36)
  line L549 (-2.5, 19.36) -> (-3.5, 19.36)
  line L550 (-3.5, 19.36) -> (-3.5, 20.36)
  line L551 (-3.5, 20.36) -> (-2.5, 20.36)
  line L552 (-2.5, 17.73) -> (-2.5, 16.73)
  line L553 (-2.5, 16.73) -> (-3.5, 16.73)
  line L554 (-3.5, 16.73) -> (-3.5, 17.73)
  line L555 (-3.5, 17.73) -> (-2.5, 17.73)
  line L556 (-2.5, 15.1) -> (-2.5, 14.1)
  line L557 (-2.5, 14.1) -> (-3.5, 14.1)
  line L558 (-3.5, 14.1) -> (-3.5, 15.1)
  line L559 (-3.5, 15.1) -> (-2.5, 15.1)
  line L560 (-2.5, 12.47) -> (-2.5, 11.47)
  line L561 (-2.5, 11.47) -> (-3.5, 11.47)
  line L562 (-3.5, 11.47) -> (-3.5, 12.47)
  line L563 (-3.5, 12.47) -> (-2.5, 12.47)
  line L564 (-2.5, 9.84) -> (-2.5, 8.84)
  line L565 (-2.5, 8.84) -> (-3.5, 8.84)
  line L566 (-3.5, 8.84) -> (-3.5, 9.84)
  line L567 (-3.5, 9.84) -> (-2.5, 9.84)
  line L568 (-2.5, 7.21) -> (-2.5, 6.21)
  line L569 (-2.5, 6.21) -> (-3.5, 6.21)
  line L570 (-3.5, 6.21) -> (-3.5, 7.21)
  line L571 (-3.5, 7.21) -> (-2.5, 7.21)
  line L572 (-2.5, 4.58) -> (-2.5, 3.58)
  line L573 (-2.5, 3.58) -> (-3.5, 3.58)
  line L574 (-3.5, 3.58) -> (-3.5, 4.58)
  line L575 (-3.5, 4.58) -> (-2.5, 4.58)
  line L576 (-2.5, 1.95) -> (-2.5, 0.95)
  line L577 (-2.5, 0.95) -> (-3.5, 0.95)
  line L578 (-3.5, 0.95) -> (-3.5, 1.95)
  line L579 (-3.5, 1.95) -> (-2.5, 1.95)
  line L580 (-2.5, -0.68) -> (-2.5, -1.68)
  line L581 (-2.5, -1.68) -> (-3.5, -1.68)
  line L582 (-3.5, -1.68) -> (-3.5, -0.68)
  line L583 (-3.5, -0.68) -> (-2.5, -0.68)
  line L584 (-2.5, -3.31) -> (-2.5, -4.31)
  line L585 (-2.5, -4.31) -> (-3.5, -4.31)
  line L586 (-3.5, -4.31) -> (-3.5, -3.31)
  line L587 (-3.5, -3.31) -> (-2.5, -3.31)
  line L588 (-2.5, -5.94) -> (-2.5, -6.94)
  line L589 (-2.5, -6.94) -> (-3.5, -6.94)
  line L590 (-3.5, -6.94) -> (-3.5, -5.94)
  line L591 (-3.5, -5.94) -> (-2.5, -5.94)
  line L592 (-2.5, -8.57) -> (-2.5, -9.57)
  line L593 (-2.5, -9.57) -> (-3.5, -9.57)
  line L594 (-3.5, -9.57) -> (-3.5, -8.57)
  line L595 (-3.5, -8.57) -> (-2.5, -8.57)
  line L596 (-2.5, -11.2) -> (-2.5, -12.2)
  line L597 (-2.5, -12.2) -> (-3.5, -12.2)
  line L598 (-3.5, -12.2) -> (-3.5, -11.2)
  line L599 (-3.5, -11.2) -> (-2.5, -11.2)
  line L600 (-2.5, -13.83) -> (-2.5, -14.83)
  line L601 (-2.5, -14.83) -> (-3.5, -14.83)
  line L602 (-3.5, -14.83) -> (-3.5, -13.83)
  line L603 (-3.5, -13.83) -> (-2.5, -13.83)
  line L604 (-2.5, -16.46) -> (-2.5, -17.46)
  line L605 (-2.5, -17.46) -> (-3.5, -17.46)
  line L606 (-3.5, -17.46) -> (-3.5, -16.46)
  line L607 (-3.5, -16.46) -> (-2.5, -16.46)
  line L608 (-2.5, -19.09) -> (-2.5, -20.09)
  line L609 (-2.5, -20.09) -> (-3.5, -20.09)
  line L610 (-3.5, -20.09) -> (-3.5, -19.09)
  line L611 (-3.5, -19.09) -> (-2.5, -19.09)
  line L612 (-2.5, -21.72) -> (-2.5, -22.72)
  line L613 (-2.5, -22.72) -> (-3.5, -22.72)
  line L614 (-3.5, -22.72) -> (-3.5, -21.72)
  line L615 (-3.5, -21.72) -> (-2.5, -21.72)
  line L616 (-2.5, -24.35) -> (-2.5, -25.35)
  line L617 (-2.5, -25.35) -> (-3.5, -25.35)
  line L618 (-3.5, -25.35) -> (-3.5, -24.35)
  line L619 (-3.5, -24.35) -> (-2.5, -24.35)
  line L620 (-2.5, -26.98) -> (-2.5, -27.98)
  line L621 (-2.5, -27.98) -> (-3.5, -27.98)
  line L622 (-3.5, -27.98) -> (-3.5, -26.98)
  line L623 (-3.5, -26.98) -> (-2.5, -26.98)
  line L624 (-2.5, -29.61) -> (-2.5, -30.61)
  line L625 (-2.5, -30.61) -> (-3.5, -30.61)
  line L626 (-3.5, -30.61) -> (-3.5, -29.61)
  line L627 (-3.5, -29.61) -> (-2.5, -29.61)
  line L628 (-2.5, -32.24) -> (-2.5, -33.24)
  line L629 (-2.5, -33.24) -> (-3.5, -33.24)
  line L630 (-3.5, -33.24) -> (-3.5, -32.24)
  line L631 (-3.5, -32.24) -> (-2.5, -32.24)
  line L632 (-2.5, -34.87) -> (-2.5, -35.87)
  line L633 (-2.5, -35.87) -> (-3.5, -35.87)
  line L634 (-3.5, -35.87) -> (-3.5, -34.87)
  line L635 (-3.5, -34.87) -> (-2.5, -34.87)
  line L636 (-2.5, -37.5) -> (-2.5, -38.5)
  line L637 (-2.5, -38.5) -> (-3.5, -38.5)
  line L638 (-3.5, -38.5) -> (-3.5, -37.5)
  line L639 (-3.5, -37.5) -> (-2.5, -37.5)
  line L640 (-1, -40.5) -> (-1, 40.5)
  line L641 (-1, 40.5) -> (-26.5, 40.5)
  line L642 (-26.5, 40.5) -> (-26.5, -40.5)
  line L643 (-26.5, -40.5) -> (-1, -40.5)
  line L644 (-24, -20.28) -> (-23, -20.28)
  line L645 (-23, -20.28) -> (-23, -21.28)
  line L646 (-23, -21.28) -> (-24, -21.28)
  line L647 (-24, -21.28) -> (-24, -20.28)
  line L648 (-24, -20.28) -> (-23, -21.28) construction
  line L649 (-23, -20.28) -> (-24, -21.28) construction
  line L650 (-26.5, -40.5) -> (-26.5, 40.5)
  point P0 (-23.5, -20.78)
  dimension "d178" = 1
  dimension "d179" = 1
  dimension "d180" = 2.5
  dimension "d181" = 3.7
  constraint horizontal L644
  constraint perpendicular L644 L645
  constraint parallel L644 L646
  constraint parallel L645 L647
  constraint coincident L648 P0
  constraint coincident L649 P0
  measures "d178" distance of L645.end L646.end
  measures "d179" distance of L644.start L646.end
  measures "d180" distance of L647 L650
  measures "d181" distance of L7 L646
extrude "Extrude30" cut sketch "Sketch30" against normal blind 1 contours L644 L645 L646 L647 bodies 1
pattern_linear "R-Pattern8" count 2 spacing 3 along (-1, 0, 0) count 5 spacing 2.63 along (0, -1, 0) of "Extrude30"
sketch "Sketch31" plane through (0, 0, 9) normal (0, 0, 1) x (-1, 0, 0)
  line L0 (-20, -9.76) -> (-20, -10.76)
  line L1 (-20, -10.76) -> (-21, -10.76)
  line L2 (-21, -10.76) -> (-21, -9.76)
  line L3 (-21, -9.76) -> (-20, -9.76)
  line L4 (-23, -9.76) -> (-23, -10.76)
  line L5 (-23, -10.76) -> (-24, -10.76)
  line L6 (-24, -10.76) -> (-24, -9.76)
  line L7 (-24, -9.76) -> (-23, -9.76)
  line L8 (-20, -12.39) -> (-20, -13.39)
  line L9 (-20, -13.39) -> (-21, -13.39)
  line L10 (-21, -13.39) -> (-21, -12.39)
  line L11 (-21, -12.39) -> (-20, -12.39)
  line L12 (-23, -12.39) -> (-23, -13.39)
  line L13 (-23, -13.39) -> (-24, -13.39)
  line L14 (-24, -13.39) -> (-24, -12.39)
  line L15 (-24, -12.39) -> (-23, -12.39)
  line L16 (-20, -15.02) -> (-20, -16.02)
  line L17 (-20, -16.02) -> (-21, -16.02)
  line L18 (-21, -16.02) -> (-21, -15.02)
  line L19 (-21, -15.02) -> (-20, -15.02)
  line L20 (-23, -15.02) -> (-23, -16.02)
  line L21 (-23, -16.02) -> (-24, -16.02)
  line L22 (-24, -16.02) -> (-24, -15.02)
  line L23 (-24, -15.02) -> (-23, -15.02)
  line L24 (-20, -17.65) -> (-20, -18.65)
  line L25 (-20, -18.65) -> (-21, -18.65)
  line L26 (-21, -18.65) -> (-21, -17.65)
  line L27 (-21, -17.65) -> (-20, -17.65)
  line L28 (-23, -17.65) -> (-23, -18.65)
  line L29 (-23, -18.65) -> (-24, -18.65)
  line L30 (-24, -18.65) -> (-24, -17.65)
  line L31 (-24, -17.65) -> (-23, -17.65)
  line L32 (-20, -20.28) -> (-20, -21.28)
  line L33 (-20, -21.28) -> (-21, -21.28)
  line L34 (-21, -21.28) -> (-21, -20.28)
  line L35 (-21, -20.28) -> (-20, -20.28)
  line L36 (-23, -20.28) -> (-23, -21.28)
  line L37 (-23, -21.28) -> (-24, -21.28)
  line L38 (-24, -21.28) -> (-24, -20.28)
  line L39 (-24, -20.28) -> (-23, -20.28)
  line L40 (-20, -24.98) -> (-20, -25.98)
  line L41 (-20, -25.98) -> (-21, -25.98)
  line L42 (-21, -25.98) -> (-21, -24.98)
  line L43 (-21, -24.98) -> (-20, -24.98)
  line L44 (-23, -24.98) -> (-23, -25.98)
  line L45 (-23, -25.98) -> (-24, -25.98)
  line L46 (-24, -25.98) -> (-24, -24.98)
  line L47 (-24, -24.98) -> (-23, -24.98)
  line L48 (-20, -27.61) -> (-20, -28.61)
  line L49 (-20, -28.61) -> (-21, -28.61)
  line L50 (-21, -28.61) -> (-21, -27.61)
  line L51 (-21, -27.61) -> (-20, -27.61)
  line L52 (-23, -27.61) -> (-23, -28.61)
  line L53 (-23, -28.61) -> (-24, -28.61)
  line L54 (-24, -28.61) -> (-24, -27.61)
  line L55 (-24, -27.61) -> (-23, -27.61)
  line L56 (-20, -30.24) -> (-20, -31.24)
  line L57 (-20, -31.24) -> (-21, -31.24)
  line L58 (-21, -31.24) -> (-21, -30.24)
  line L59 (-21, -30.24) -> (-20, -30.24)
  line L60 (-23, -30.24) -> (-23, -31.24)
  line L61 (-23, -31.24) -> (-24, -31.24)
  line L62 (-24, -31.24) -> (-24, -30.24)
  line L63 (-24, -30.24) -> (-23, -30.24)
  line L64 (-20, -32.87) -> (-20, -33.87)
  line L65 (-20, -33.87) -> (-21, -33.87)
  line L66 (-21, -33.87) -> (-21, -32.87)
  line L67 (-21, -32.87) -> (-20, -32.87)
  line L68 (-23, -32.87) -> (-23, -33.87)
  line L69 (-23, -33.87) -> (-24, -33.87)
  line L70 (-24, -33.87) -> (-24, -32.87)
  line L71 (-24, -32.87) -> (-23, -32.87)
  line L72 (-20, -35.5) -> (-20, -36.5)
  line L73 (-20, -36.5) -> (-21, -36.5)
  line L74 (-21, -36.5) -> (-21, -35.5)
  line L75 (-21, -35.5) -> (-20, -35.5)
  line L76 (-23, -35.5) -> (-23, -36.5)
  line L77 (-23, -36.5) -> (-24, -36.5)
  line L78 (-24, -36.5) -> (-24, -35.5)
  line L79 (-24, -35.5) -> (-23, -35.5)
  line L80 (-13.7, 38.77) -> (-13.7, 37.77)
  line L81 (-13.7, 37.77) -> (-14.7, 37.77)
  line L82 (-14.7, 37.77) -> (-14.7, 38.77)
  line L83 (-14.7, 38.77) -> (-13.7, 38.77)
  line L84 (-13.7, 36.14) -> (-13.7, 35.14)
  line L85 (-13.7, 35.14) -> (-14.7, 35.14)
  line L86 (-14.7, 35.14) -> (-14.7, 36.14)
  line L87 (-14.7, 36.14) -> (-13.7, 36.14)
  line L88 (-13.7, 33.51) -> (-13.7, 32.51)
  line L89 (-13.7, 32.51) -> (-14.7, 32.51)
  line L90 (-14.7, 32.51) -> (-14.7, 33.51)
  line L91 (-14.7, 33.51) -> (-13.7, 33.51)
  line L92 (-13.7, 30.88) -> (-13.7, 29.88)
  line L93 (-13.7, 29.88) -> (-14.7, 29.88)
  line L94 (-14.7, 29.88) -> (-14.7, 30.88)
  line L95 (-14.7, 30.88) -> (-13.7, 30.88)
  line L96 (-13.7, 28.25) -> (-13.7, 27.25)
  line L97 (-13.7, 27.25) -> (-14.7, 27.25)
  line L98 (-14.7, 27.25) -> (-14.7, 28.25)
  line L99 (-14.7, 28.25) -> (-13.7, 28.25)
  line L100 (-13.7, 25.62) -> (-13.7, 24.62)
  line L101 (-13.7, 24.62) -> (-14.7, 24.62)
  line L102 (-14.7, 24.62) -> (-14.7, 25.62)
  line L103 (-14.7, 25.62) -> (-13.7, 25.62)
  line L104 (-13.7, 22.99) -> (-13.7, 21.99)
  line L105 (-13.7, 21.99) -> (-14.7, 21.99)
  line L106 (-14.7, 21.99) -> (-14.7, 22.99)
  line L107 (-14.7, 22.99) -> (-13.7, 22.99)
  line L108 (-13.7, 20.36) -> (-13.7, 19.36)
  line L109 (-13.7, 19.36) -> (-14.7, 19.36)
  line L110 (-14.7, 19.36) -> (-14.7, 20.36)
  line L111 (-14.7, 20.36) -> (-13.7, 20.36)
  line L112 (-13.7, 17.73) -> (-13.7, 16.73)
  line L113 (-13.7, 16.73) -> (-14.7, 16.73)
  line L114 (-14.7, 16.73) -> (-14.7, 17.73)
  line L115 (-14.7, 17.73) -> (-13.7, 17.73)
  line L116 (-13.7, 15.1) -> (-13.7, 14.1)
  line L117 (-13.7, 14.1) -> (-14.7, 14.1)
  line L118 (-14.7, 14.1) -> (-14.7, 15.1)
  line L119 (-14.7, 15.1) -> (-13.7, 15.1)
  line L120 (-13.7, 12.47) -> (-13.7, 11.47)
  line L121 (-13.7, 11.47) -> (-14.7, 11.47)
  line L122 (-14.7, 11.47) -> (-14.7, 12.47)
  line L123 (-14.7, 12.47) -> (-13.7, 12.47)
  line L124 (-13.7, 9.84) -> (-13.7, 8.84)
  line L125 (-13.7, 8.84) -> (-14.7, 8.84)
  line L126 (-14.7, 8.84) -> (-14.7, 9.84)
  line L127 (-14.7, 9.84) -> (-13.7, 9.84)
  line L128 (-13.7, 7.21) -> (-13.7, 6.21)
  line L129 (-13.7, 6.21) -> (-14.7, 6.21)
  line L130 (-14.7, 6.21) -> (-14.7, 7.21)
  line L131 (-14.7, 7.21) -> (-13.7, 7.21)
  line L132 (-13.7, 4.58) -> (-13.7, 3.58)
  line L133 (-13.7, 3.58) -> (-14.7, 3.58)
  line L134 (-14.7, 3.58) -> (-14.7, 4.58)
  line L135 (-14.7, 4.58) -> (-13.7, 4.58)
  line L136 (-13.7, 1.95) -> (-13.7, 0.95)
  line L137 (-13.7, 0.95) -> (-14.7, 0.95)
  line L138 (-14.7, 0.95) -> (-14.7, 1.95)
  line L139 (-14.7, 1.95) -> (-13.7, 1.95)
  line L140 (-13.7, -0.68) -> (-13.7, -1.68)
  line L141 (-13.7, -1.68) -> (-14.7, -1.68)
  line L142 (-14.7, -1.68) -> (-14.7, -0.68)
  line L143 (-14.7, -0.68) -> (-13.7, -0.68)
  line L144 (-13.7, -3.31) -> (-13.7, -4.31)
  line L145 (-13.7, -4.31) -> (-14.7, -4.31)
  line L146 (-14.7, -4.31) -> (-14.7, -3.31)
  line L147 (-14.7, -3.31) -> (-13.7, -3.31)
  line L148 (-13.7, -5.94) -> (-13.7, -6.94)
  line L149 (-13.7, -6.94) -> (-14.7, -6.94)
  line L150 (-14.7, -6.94) -> (-14.7, -5.94)
  line L151 (-14.7, -5.94) -> (-13.7, -5.94)
  line L152 (-13.7, -8.57) -> (-13.7, -9.57)
  line L153 (-13.7, -9.57) -> (-14.7, -9.57)
  line L154 (-14.7, -9.57) -> (-14.7, -8.57)
  line L155 (-14.7, -8.57) -> (-13.7, -8.57)
  line L156 (-13.7, -11.2) -> (-13.7, -12.2)
  line L157 (-13.7, -12.2) -> (-14.7, -12.2)
  line L158 (-14.7, -12.2) -> (-14.7, -11.2)
  line L159 (-14.7, -11.2) -> (-13.7, -11.2)
  line L160 (-13.7, -13.83) -> (-13.7, -14.83)
  line L161 (-13.7, -14.83) -> (-14.7, -14.83)
  line L162 (-14.7, -14.83) -> (-14.7, -13.83)
  line L163 (-14.7, -13.83) -> (-13.7, -13.83)
  line L164 (-13.7, -16.46) -> (-13.7, -17.46)
  line L165 (-13.7, -17.46) -> (-14.7, -17.46)
  line L166 (-14.7, -17.46) -> (-14.7, -16.46)
  line L167 (-14.7, -16.46) -> (-13.7, -16.46)
  line L168 (-13.7, -19.09) -> (-13.7, -20.09)
  line L169 (-13.7, -20.09) -> (-14.7, -20.09)
  line L170 (-14.7, -20.09) -> (-14.7, -19.09)
  line L171 (-14.7, -19.09) -> (-13.7, -19.09)
  line L172 (-13.7, -21.72) -> (-13.7, -22.72)
  line L173 (-13.7, -22.72) -> (-14.7, -22.72)
  line L174 (-14.7, -22.72) -> (-14.7, -21.72)
  line L175 (-14.7, -21.72) -> (-13.7, -21.72)
  line L176 (-13.7, -24.35) -> (-13.7, -25.35)
  line L177 (-13.7, -25.35) -> (-14.7, -25.35)
  line L178 (-14.7, -25.35) -> (-14.7, -24.35)
  line L179 (-14.7, -24.35) -> (-13.7, -24.35)
  line L180 (-13.7, -26.98) -> (-13.7, -27.98)
  line L181 (-13.7, -27.98) -> (-14.7, -27.98)
  line L182 (-14.7, -27.98) -> (-14.7, -26.98)
  line L183 (-14.7, -26.98) -> (-13.7, -26.98)
  line L184 (-13.7, -29.61) -> (-13.7, -30.61)
  line L185 (-13.7, -30.61) -> (-14.7, -30.61)
  line L186 (-14.7, -30.61) -> (-14.7, -29.61)
  line L187 (-14.7, -29.61) -> (-13.7, -29.61)
  line L188 (-13.7, -32.24) -> (-13.7, -33.24)
  line L189 (-13.7, -33.24) -> (-14.7, -33.24)
  line L190 (-14.7, -33.24) -> (-14.7, -32.24)
  line L191 (-14.7, -32.24) -> (-13.7, -32.24)
  line L192 (-13.7, -34.87) -> (-13.7, -35.87)
  line L193 (-13.7, -35.87) -> (-14.7, -35.87)
  line L194 (-14.7, -35.87) -> (-14.7, -34.87)
  line L195 (-14.7, -34.87) -> (-13.7, -34.87)
  line L196 (-13.7, -37.5) -> (-13.7, -38.5)
  line L197 (-13.7, -38.5) -> (-14.7, -38.5)
  line L198 (-14.7, -38.5) -> (-14.7, -37.5)
  line L199 (-14.7, -37.5) -> (-13.7, -37.5)
  line L200 (-10.9, 38.77) -> (-10.9, 37.77)
  line L201 (-10.9, 37.77) -> (-11.9, 37.77)
  line L202 (-11.9, 37.77) -> (-11.9, 38.77)
  line L203 (-11.9, 38.77) -> (-10.9, 38.77)
  line L204 (-10.9, 36.14) -> (-10.9, 35.14)
  line L205 (-10.9, 35.14) -> (-11.9, 35.14)
  line L206 (-11.9, 35.14) -> (-11.9, 36.14)
  line L207 (-11.9, 36.14) -> (-10.9, 36.14)
  line L208 (-10.9, 33.51) -> (-10.9, 32.51)
  line L209 (-10.9, 32.51) -> (-11.9, 32.51)
  line L210 (-11.9, 32.51) -> (-11.9, 33.51)
  line L211 (-11.9, 33.51) -> (-10.9, 33.51)
  line L212 (-10.9, 30.88) -> (-10.9, 29.88)
  line L213 (-10.9, 29.88) -> (-11.9, 29.88)
  line L214 (-11.9, 29.88) -> (-11.9, 30.88)
  line L215 (-11.9, 30.88) -> (-10.9, 30.88)
  line L216 (-10.9, 28.25) -> (-10.9, 27.25)
  line L217 (-10.9, 27.25) -> (-11.9, 27.25)
  line L218 (-11.9, 27.25) -> (-11.9, 28.25)
  line L219 (-11.9, 28.25) -> (-10.9, 28.25)
  line L220 (-10.9, 25.62) -> (-10.9, 24.62)
  line L221 (-10.9, 24.62) -> (-11.9, 24.62)
  line L222 (-11.9, 24.62) -> (-11.9, 25.62)
  line L223 (-11.9, 25.62) -> (-10.9, 25.62)
  line L224 (-10.9, 22.99) -> (-10.9, 21.99)
  line L225 (-10.9, 21.99) -> (-11.9, 21.99)
  line L226 (-11.9, 21.99) -> (-11.9, 22.99)
  line L227 (-11.9, 22.99) -> (-10.9, 22.99)
  line L228 (-10.9, 20.36) -> (-10.9, 19.36)
  line L229 (-10.9, 19.36) -> (-11.9, 19.36)
  line L230 (-11.9, 19.36) -> (-11.9, 20.36)
  line L231 (-11.9, 20.36) -> (-10.9, 20.36)
  line L232 (-10.9, 17.73) -> (-10.9, 16.73)
  line L233 (-10.9, 16.73) -> (-11.9, 16.73)
  line L234 (-11.9, 16.73) -> (-11.9, 17.73)
  line L235 (-11.9, 17.73) -> (-10.9, 17.73)
  line L236 (-10.9, 15.1) -> (-10.9, 14.1)
  line L237 (-10.9, 14.1) -> (-11.9, 14.1)
  line L238 (-11.9, 14.1) -> (-11.9, 15.1)
  line L239 (-11.9, 15.1) -> (-10.9, 15.1)
  line L240 (-10.9, 12.47) -> (-10.9, 11.47)
  line L241 (-10.9, 11.47) -> (-11.9, 11.47)
  line L242 (-11.9, 11.47) -> (-11.9, 12.47)
  line L243 (-11.9, 12.47) -> (-10.9, 12.47)
  line L244 (-10.9, 9.84) -> (-10.9, 8.84)
  line L245 (-10.9, 8.84) -> (-11.9, 8.84)
  line L246 (-11.9, 8.84) -> (-11.9, 9.84)
  line L247 (-11.9, 9.84) -> (-10.9, 9.84)
  line L248 (-10.9, 7.21) -> (-10.9, 6.21)
  line L249 (-10.9, 6.21) -> (-11.9, 6.21)
  line L250 (-11.9, 6.21) -> (-11.9, 7.21)
  line L251 (-11.9, 7.21) -> (-10.9, 7.21)
  line L252 (-10.9, 4.58) -> (-10.9, 3.58)
  line L253 (-10.9, 3.58) -> (-11.9, 3.58)
  line L254 (-11.9, 3.58) -> (-11.9, 4.58)
  line L255 (-11.9, 4.58) -> (-10.9, 4.58)
  line L256 (-10.9, 1.95) -> (-10.9, 0.95)
  line L257 (-10.9, 0.95) -> (-11.9, 0.95)
  line L258 (-11.9, 0.95) -> (-11.9, 1.95)
  line L259 (-11.9, 1.95) -> (-10.9, 1.95)
  line L260 (-10.9, -0.68) -> (-10.9, -1.68)
  line L261 (-10.9, -1.68) -> (-11.9, -1.68)
  line L262 (-11.9, -1.68) -> (-11.9, -0.68)
  line L263 (-11.9, -0.68) -> (-10.9, -0.68)
  line L264 (-10.9, -3.31) -> (-10.9, -4.31)
  line L265 (-10.9, -4.31) -> (-11.9, -4.31)
  line L266 (-11.9, -4.31) -> (-11.9, -3.31)
  line L267 (-11.9, -3.31) -> (-10.9, -3.31)
  line L268 (-10.9, -5.94) -> (-10.9, -6.94)
  line L269 (-10.9, -6.94) -> (-11.9, -6.94)
  line L270 (-11.9, -6.94) -> (-11.9, -5.94)
  line L271 (-11.9, -5.94) -> (-10.9, -5.94)
  line L272 (-10.9, -8.57) -> (-10.9, -9.57)
  line L273 (-10.9, -9.57) -> (-11.9, -9.57)
  line L274 (-11.9, -9.57) -> (-11.9, -8.57)
  line L275 (-11.9, -8.57) -> (-10.9, -8.57)
  line L276 (-10.9, -11.2) -> (-10.9, -12.2)
  line L277 (-10.9, -12.2) -> (-11.9, -12.2)
  line L278 (-11.9, -12.2) -> (-11.9, -11.2)
  line L279 (-11.9, -11.2) -> (-10.9, -11.2)
  line L280 (-10.9, -13.83) -> (-10.9, -14.83)
  line L281 (-10.9, -14.83) -> (-11.9, -14.83)
  line L282 (-11.9, -14.83) -> (-11.9, -13.83)
  line L283 (-11.9, -13.83) -> (-10.9, -13.83)
  line L284 (-10.9, -16.46) -> (-10.9, -17.46)
  line L285 (-10.9, -17.46) -> (-11.9, -17.46)
  line L286 (-11.9, -17.46) -> (-11.9, -16.46)
  line L287 (-11.9, -16.46) -> (-10.9, -16.46)
  line L288 (-10.9, -19.09) -> (-10.9, -20.09)
  line L289 (-10.9, -20.09) -> (-11.9, -20.09)
  line L290 (-11.9, -20.09) -> (-11.9, -19.09)
  line L291 (-11.9, -19.09) -> (-10.9, -19.09)
  line L292 (-10.9, -21.72) -> (-10.9, -22.72)
  line L293 (-10.9, -22.72) -> (-11.9, -22.72)
  line L294 (-11.9, -22.72) -> (-11.9, -21.72)
  line L295 (-11.9, -21.72) -> (-10.9, -21.72)
  line L296 (-10.9, -24.35) -> (-10.9, -25.35)
  line L297 (-10.9, -25.35) -> (-11.9, -25.35)
  line L298 (-11.9, -25.35) -> (-11.9, -24.35)
  line L299 (-11.9, -24.35) -> (-10.9, -24.35)
  line L300 (-10.9, -26.98) -> (-10.9, -27.98)
  line L301 (-10.9, -27.98) -> (-11.9, -27.98)
  line L302 (-11.9, -27.98) -> (-11.9, -26.98)
  line L303 (-11.9, -26.98) -> (-10.9, -26.98)
  line L304 (-10.9, -29.61) -> (-10.9, -30.61)
  line L305 (-10.9, -30.61) -> (-11.9, -30.61)
  line L306 (-11.9, -30.61) -> (-11.9, -29.61)
  line L307 (-11.9, -29.61) -> (-10.9, -29.61)
  line L308 (-10.9, -32.24) -> (-10.9, -33.24)
  line L309 (-10.9, -33.24) -> (-11.9, -33.24)
  line L310 (-11.9, -33.24) -> (-11.9, -32.24)
  line L311 (-11.9, -32.24) -> (-10.9, -32.24)
  line L312 (-10.9, -34.87) -> (-10.9, -35.87)
  line L313 (-10.9, -35.87) -> (-11.9, -35.87)
  line L314 (-11.9, -35.87) -> (-11.9, -34.87)
  line L315 (-11.9, -34.87) -> (-10.9, -34.87)
  line L316 (-10.9, -37.5) -> (-10.9, -38.5)
  line L317 (-10.9, -38.5) -> (-11.9, -38.5)
  line L318 (-11.9, -38.5) -> (-11.9, -37.5)
  line L319 (-11.9, -37.5) -> (-10.9, -37.5)
  line L320 (-8.1, 38.77) -> (-8.1, 37.77)
  line L321 (-8.1, 37.77) -> (-9.1, 37.77)
  line L322 (-9.1, 37.77) -> (-9.1, 38.77)
  line L323 (-9.1, 38.77) -> (-8.1, 38.77)
  line L324 (-8.1, 36.14) -> (-8.1, 35.14)
  line L325 (-8.1, 35.14) -> (-9.1, 35.14)
  line L326 (-9.1, 35.14) -> (-9.1, 36.14)
  line L327 (-9.1, 36.14) -> (-8.1, 36.14)
  line L328 (-8.1, 33.51) -> (-8.1, 32.51)
  line L329 (-8.1, 32.51) -> (-9.1, 32.51)
  line L330 (-9.1, 32.51) -> (-9.1, 33.51)
  line L331 (-9.1, 33.51) -> (-8.1, 33.51)
  line L332 (-8.1, 30.88) -> (-8.1, 29.88)
  line L333 (-8.1, 29.88) -> (-9.1, 29.88)
  line L334 (-9.1, 29.88) -> (-9.1, 30.88)
  line L335 (-9.1, 30.88) -> (-8.1, 30.88)
  line L336 (-8.1, 28.25) -> (-8.1, 27.25)
  line L337 (-8.1, 27.25) -> (-9.1, 27.25)
  line L338 (-9.1, 27.25) -> (-9.1, 28.25)
  line L339 (-9.1, 28.25) -> (-8.1, 28.25)
  line L340 (-8.1, 25.62) -> (-8.1, 24.62)
  line L341 (-8.1, 24.62) -> (-9.1, 24.62)
  line L342 (-9.1, 24.62) -> (-9.1, 25.62)
  line L343 (-9.1, 25.62) -> (-8.1, 25.62)
  line L344 (-8.1, 22.99) -> (-8.1, 21.99)
  line L345 (-8.1, 21.99) -> (-9.1, 21.99)
  line L346 (-9.1, 21.99) -> (-9.1, 22.99)
  line L347 (-9.1, 22.99) -> (-8.1, 22.99)
  line L348 (-8.1, 20.36) -> (-8.1, 19.36)
  line L349 (-8.1, 19.36) -> (-9.1, 19.36)
  line L350 (-9.1, 19.36) -> (-9.1, 20.36)
  line L351 (-9.1, 20.36) -> (-8.1, 20.36)
  line L352 (-8.1, 17.73) -> (-8.1, 16.73)
  line L353 (-8.1, 16.73) -> (-9.1, 16.73)
  line L354 (-9.1, 16.73) -> (-9.1, 17.73)
  line L355 (-9.1, 17.73) -> (-8.1, 17.73)
  line L356 (-8.1, 15.1) -> (-8.1, 14.1)
  line L357 (-8.1, 14.1) -> (-9.1, 14.1)
  line L358 (-9.1, 14.1) -> (-9.1, 15.1)
  line L359 (-9.1, 15.1) -> (-8.1, 15.1)
  line L360 (-8.1, 12.47) -> (-8.1, 11.47)
  line L361 (-8.1, 11.47) -> (-9.1, 11.47)
  line L362 (-9.1, 11.47) -> (-9.1, 12.47)
  line L363 (-9.1, 12.47) -> (-8.1, 12.47)
  line L364 (-8.1, 9.84) -> (-8.1, 8.84)
  line L365 (-8.1, 8.84) -> (-9.1, 8.84)
  line L366 (-9.1, 8.84) -> (-9.1, 9.84)
  line L367 (-9.1, 9.84) -> (-8.1, 9.84)
  line L368 (-8.1, 7.21) -> (-8.1, 6.21)
  line L369 (-8.1, 6.21) -> (-9.1, 6.21)
  line L370 (-9.1, 6.21) -> (-9.1, 7.21)
  line L371 (-9.1, 7.21) -> (-8.1, 7.21)
  line L372 (-8.1, 4.58) -> (-8.1, 3.58)
  line L373 (-8.1, 3.58) -> (-9.1, 3.58)
  line L374 (-9.1, 3.58) -> (-9.1, 4.58)
  line L375 (-9.1, 4.58) -> (-8.1, 4.58)
  line L376 (-8.1, 1.95) -> (-8.1, 0.95)
  line L377 (-8.1, 0.95) -> (-9.1, 0.95)
  line L378 (-9.1, 0.95) -> (-9.1, 1.95)
  line L379 (-9.1, 1.95) -> (-8.1, 1.95)
  line L380 (-8.1, -0.68) -> (-8.1, -1.68)
  line L381 (-8.1, -1.68) -> (-9.1, -1.68)
  line L382 (-9.1, -1.68) -> (-9.1, -0.68)
  line L383 (-9.1, -0.68) -> (-8.1, -0.68)
  line L384 (-8.1, -3.31) -> (-8.1, -4.31)
  line L385 (-8.1, -4.31) -> (-9.1, -4.31)
  line L386 (-9.1, -4.31) -> (-9.1, -3.31)
  line L387 (-9.1, -3.31) -> (-8.1, -3.31)
  line L388 (-8.1, -5.94) -> (-8.1, -6.94)
  line L389 (-8.1, -6.94) -> (-9.1, -6.94)
  line L390 (-9.1, -6.94) -> (-9.1, -5.94)
  line L391 (-9.1, -5.94) -> (-8.1, -5.94)
  line L392 (-8.1, -8.57) -> (-8.1, -9.57)
  line L393 (-8.1, -9.57) -> (-9.1, -9.57)
  line L394 (-9.1, -9.57) -> (-9.1, -8.57)
  line L395 (-9.1, -8.57) -> (-8.1, -8.57)
  line L396 (-8.1, -11.2) -> (-8.1, -12.2)
  line L397 (-8.1, -12.2) -> (-9.1, -12.2)
  line L398 (-9.1, -12.2) -> (-9.1, -11.2)
  line L399 (-9.1, -11.2) -> (-8.1, -11.2)
  line L400 (-8.1, -13.83) -> (-8.1, -14.83)
  line L401 (-8.1, -14.83) -> (-9.1, -14.83)
  line L402 (-9.1, -14.83) -> (-9.1, -13.83)
  line L403 (-9.1, -13.83) -> (-8.1, -13.83)
  line L404 (-8.1, -16.46) -> (-8.1, -17.46)
  line L405 (-8.1, -17.46) -> (-9.1, -17.46)
  line L406 (-9.1, -17.46) -> (-9.1, -16.46)
  line L407 (-9.1, -16.46) -> (-8.1, -16.46)
  line L408 (-8.1, -19.09) -> (-8.1, -20.09)
  line L409 (-8.1, -20.09) -> (-9.1, -20.09)
  line L410 (-9.1, -20.09) -> (-9.1, -19.09)
  line L411 (-9.1, -19.09) -> (-8.1, -19.09)
  line L412 (-8.1, -21.72) -> (-8.1, -22.72)
  line L413 (-8.1, -22.72) -> (-9.1, -22.72)
  line L414 (-9.1, -22.72) -> (-9.1, -21.72)
  line L415 (-9.1, -21.72) -> (-8.1, -21.72)
  line L416 (-8.1, -24.35) -> (-8.1, -25.35)
  line L417 (-8.1, -25.35) -> (-9.1, -25.35)
  line L418 (-9.1, -25.35) -> (-9.1, -24.35)
  line L419 (-9.1, -24.35) -> (-8.1, -24.35)
  line L420 (-8.1, -26.98) -> (-8.1, -27.98)
  line L421 (-8.1, -27.98) -> (-9.1, -27.98)
  line L422 (-9.1, -27.98) -> (-9.1, -26.98)
  line L423 (-9.1, -26.98) -> (-8.1, -26.98)
  line L424 (-8.1, -29.61) -> (-8.1, -30.61)
  line L425 (-8.1, -30.61) -> (-9.1, -30.61)
  line L426 (-9.1, -30.61) -> (-9.1, -29.61)
  line L427 (-9.1, -29.61) -> (-8.1, -29.61)
  line L428 (-8.1, -32.24) -> (-8.1, -33.24)
  line L429 (-8.1, -33.24) -> (-9.1, -33.24)
  line L430 (-9.1, -33.24) -> (-9.1, -32.24)
  line L431 (-9.1, -32.24) -> (-8.1, -32.24)
  line L432 (-8.1, -34.87) -> (-8.1, -35.87)
  line L433 (-8.1, -35.87) -> (-9.1, -35.87)
  line L434 (-9.1, -35.87) -> (-9.1, -34.87)
  line L435 (-9.1, -34.87) -> (-8.1, -34.87)
  line L436 (-8.1, -37.5) -> (-8.1, -38.5)
  line L437 (-8.1, -38.5) -> (-9.1, -38.5)
  line L438 (-9.1, -38.5) -> (-9.1, -37.5)
  line L439 (-9.1, -37.5) -> (-8.1, -37.5)
  line L440 (-5.3, 38.77) -> (-5.3, 37.77)
  line L441 (-5.3, 37.77) -> (-6.3, 37.77)
  line L442 (-6.3, 37.77) -> (-6.3, 38.77)
  line L443 (-6.3, 38.77) -> (-5.3, 38.77)
  line L444 (-5.3, 36.14) -> (-5.3, 35.14)
  line L445 (-5.3, 35.14) -> (-6.3, 35.14)
  line L446 (-6.3, 35.14) -> (-6.3, 36.14)
  line L447 (-6.3, 36.14) -> (-5.3, 36.14)
  line L448 (-5.3, 33.51) -> (-5.3, 32.51)
  line L449 (-5.3, 32.51) -> (-6.3, 32.51)
  line L450 (-6.3, 32.51) -> (-6.3, 33.51)
  line L451 (-6.3, 33.51) -> (-5.3, 33.51)
  line L452 (-5.3, 30.88) -> (-5.3, 29.88)
  line L453 (-5.3, 29.88) -> (-6.3, 29.88)
  line L454 (-6.3, 29.88) -> (-6.3, 30.88)
  line L455 (-6.3, 30.88) -> (-5.3, 30.88)
  line L456 (-5.3, 28.25) -> (-5.3, 27.25)
  line L457 (-5.3, 27.25) -> (-6.3, 27.25)
  line L458 (-6.3, 27.25) -> (-6.3, 28.25)
  line L459 (-6.3, 28.25) -> (-5.3, 28.25)
  line L460 (-5.3, 25.62) -> (-5.3, 24.62)
  line L461 (-5.3, 24.62) -> (-6.3, 24.62)
  line L462 (-6.3, 24.62) -> (-6.3, 25.62)
  line L463 (-6.3, 25.62) -> (-5.3, 25.62)
  line L464 (-5.3, 22.99) -> (-5.3, 21.99)
  line L465 (-5.3, 21.99) -> (-6.3, 21.99)
  line L466 (-6.3, 21.99) -> (-6.3, 22.99)